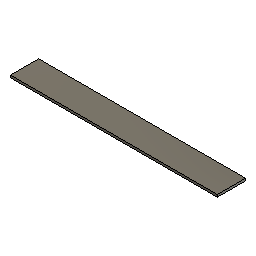
Gearbox_supportplateF v3 (Autodesk Fusion 360 design; units mm, degrees)
Autodesk Fusion 360 part; units mm, degrees
sketch "Sketch1" plane through (0, 0, 0) normal (0, 1, 0) x (1, 0, 0)
  line L0 (0, 0) -> (176, 0)
  line L1 (176, 0) -> (176, 24)
  line L2 (176, 24) -> (0, 24)
  line L3 (0, 24) -> (0, 0)
  dimension "d1" = 176
  dimension "d2" = 24
  constraint horizontal L0
  constraint vertical L1
  constraint horizontal L2
  constraint vertical L3
  constraint coincident L0.start L3.end
  measures "d1" distance of L0.start L0.end
  measures "d2" distance of L0.start L2.end
extrude "Extrude1" add sketch "Sketch1" along normal blind 2
